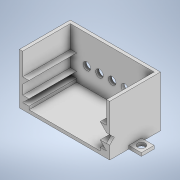
# Autodesk Inventor part: PCB_Case02
Saved by Autodesk Inventor 2021 (Build 250183000, 183)
## iProperties
Created: 2021-02-15
Part Number: PCB_Case02
Material: Generic
Document SubType Name: Modeling
Designer: Ryan
Density: 1 g/cm^3
Appearance: Default
Author: Ryan
Autodesk Inventor part; units mm, degrees
ref_plane "YZ Plane" through (0, 0, 0) normal (1, 0, 0) x (0, 1, 0)
ref_plane "XZ Plane" through (0, 0, 0) normal (0, 1, 0) x (-1, 0, 0)
ref_plane "XY Plane" through (0, 0, 0) normal (0, 0, 1) x (1, 0, 0)
sketch "Sketch1" plane through (0, 0, 0) normal (0, 1, 0) x (-1, 0, 0)
  line L0 (45.085, 25.4) -> (-45.085, 25.4)
  line L1 (-45.085, 25.4) -> (-45.085, -25.4)
  line L2 (-45.085, -25.4) -> (45.085, -25.4)
  line L3 (45.085, -25.4) -> (45.085, 25.4)
  point P0 (0, 0)
  dimension "d0" = 90.17
  dimension "d1" = 45.085
  dimension "d2" = 50.8
  dimension "d3" = 25.4
  constraints: 8 end point, 2 parallel, 1 horizontal, 1 perpendicular
  measures "d0" distance of L0.start L0.end
  measures "d1" distance from line of point (0, 0) L3
  measures "d2" distance of L0.end L1.end
  measures "d3" distance from line of point (0, 0) L2
extrude "Extrusion1" add sketch "Sketch1" along normal blind 50.8
sketch "Sketch2" plane through (0, 0, 0) normal (0, 1, 0) x (-1, 0, 0)
  line L0 (45.085, -25.4) -> (45.085, 25.4) projected
  line L1 (45.085, 6.35) -> (57.785, 6.35)
  line L2 (57.785, 6.35) -> (57.785, -6.35)
  line L3 (57.785, -6.35) -> (45.085, -6.35)
  line L4 (45.085, -6.35) -> (45.085, 6.35)
  line L5 (-45.085, 25.4) -> (-45.085, -25.4) projected
  line L6 (-45.085, -6.35) -> (-57.785, -6.35)
  line L7 (-57.785, -6.35) -> (-57.785, 6.35)
  line L8 (-57.785, 6.35) -> (-45.085, 6.35)
  line L9 (-45.085, 6.35) -> (-45.085, -6.35)
  circle A0 centre (51.435, 0) radius 3.81
  circle A1 centre (-51.435, 0) radius 3.81
  line L10 (51.435, 0) -> (51.435, -6.35) construction
  point P0 (0, 0)
  point P1 (-45.085, 6.35)
  point P2 (45.085, -6.35)
  dimension "d6" = 12.7
  dimension "d7" = 12.7
  dimension "d8" = 6.35
  dimension "d9" = 7.62
  dimension "d34" = 6.35
  dimension "d35" = 6.35
  dimension "d37" = 6.35
  constraints: 18 end point, 4 parallel, 2 centre point, 2 equal length, 2 horizontal, 2 perpendicular, 2 point on line, 1 collinear, 1 equal radius, 1 midpoint
  measures "d6" distance of L7.end L8.end
  measures "d7" distance of L6.end L7.end
  measures "d8" distance from line of point (0, 0) L6
  measures "d9" diameter of A0
  measures "d34" distance from line of L7 A1.centre
  measures "d35" distance from line of L6 A1.centre
  measures "d37" distance from line of L2 L10.start
extrude "Extrusion2" add sketch "Sketch2" along normal blind 3.175
sketch "Sketch4" plane through (-45.085, 0, 25.4) normal (0, 0, 1) x (1, 0, 0)
  line L0 (9.525, 3.175) -> (80.645, 3.175)
  line L1 (90.17, 0) -> (90.17, 50.8) projected
  line L2 (0, 50.8) -> (90.17, 50.8) projected
  line L3 (0, 0) -> (90.17, 0) projected
  line L4 (3.175, 40.8121) -> (3.175, 50.8)
  line L5 (90.17, 50.8) -> (0, 50.8) projected
  circle A0 centre (13.335, 40.8121) radius 2.5681 construction
  circle A1 centre (29.21, 40.8121) radius 2.5681 construction
  circle A2 centre (45.085, 40.8121) radius 2.6318 construction
  circle A3 centre (60.96, 40.8121) radius 2.9599 construction
  circle A4 centre (76.835, 40.8121) radius 2.9663 construction
  line L6 (3.175, 40.8121) -> (13.335, 40.8121) construction
  line L7 (13.335, 40.8121) -> (29.21, 40.8121) construction
  line L8 (29.21, 40.8121) -> (45.085, 40.8121) construction
  line L9 (45.085, 40.8121) -> (60.96, 40.8121) construction
  line L10 (60.96, 40.8121) -> (76.835, 40.8121) construction
  line L11 (76.835, 40.8121) -> (86.995, 40.8121) construction
  line L12 (3.175, 6.35) -> (9.525, 12.7)
  line L13 (9.525, 12.7) -> (3.175, 12.7)
  line L14 (3.175, 22.225) -> (9.525, 28.575)
  line L15 (9.525, 28.575) -> (3.175, 28.575)
  line L16 (45.085, 3.175) -> (45.085, 50.8) construction
  line L17 (3.175, 22.225) -> (3.175, 12.7)
  line L18 (0, 0) -> (0, 50.8) projected
  line L19 (90.17, 0) -> (0, 0) projected
  line L20 (3.175, 6.35) -> (9.525, 6.35)
  line L21 (9.525, 6.35) -> (9.525, 3.175)
  line L22 (86.995, 6.35) -> (80.645, 6.35)
  line L23 (80.645, 6.35) -> (80.645, 3.175)
  line L24 (3.175, 28.575) -> (3.175, 40.8121)
  line L25 (86.995, 12.7) -> (86.995, 6.35)
  line L26 (86.995, 6.35) -> (80.645, 12.7)
  line L27 (80.645, 12.7) -> (86.995, 12.7)
  line L28 (86.995, 22.225) -> (80.645, 28.575)
  line L29 (80.645, 28.575) -> (86.995, 28.575)
  line L30 (86.995, 22.225) -> (86.995, 12.7)
  line L31 (86.995, 28.575) -> (86.995, 40.8121)
  line L32 (86.995, 40.8121) -> (86.995, 50.8)
  line L33 (90.17, 0) -> (90.17, 50.8) projected
  point P0 (45.085, 0)
  point P1 (3.175, 6.35)
  dimension "d15" = 3.175
  dimension "d19" = 15.875
  dimension "d22" = 6.35
  dimension "d23" = 9.525
  dimension "d25" = 6.35
  dimension "d26" = 25.4
  dimension "d39" = 6.35
  dimension "d40" = 6.35
  dimension "d41" = 3.175
  dimension "d42" = 3.175
  constraints: 54 end point, 9 collinear, 6 perpendicular, 5 centre point, 5 symmetric about line, 3 horizontal, 3 point on line, 2 midpoint, 2 parallel
  measures "d15" distance between parallel lines of L3 L0
  measures "d19" distance of L6.end L7.end
  measures "d22" distance of L13.end L12.end
  measures "d23" distance between parallel lines of L0 L13
  measures "d25" distance of L14.end L15.end
  measures "d26" distance between parallel lines of L0 L15
  measures "d39" distance of L20.start L20.end
  measures "d40" distance of L22.start L22.end
  measures "d41" distance of L0.start L20.end
  measures "d42" distance of L0.end L22.end
extrude "Extrusion3" cut sketch "Sketch4" against normal blind 47.625 contours L21 L20 L12 L13 L17 L14 L15 L24 L4 L2 L32 L31 L29 L28 L30 L27 L26 L22 L23 L0
sketch "Sketch5" plane through (-45.085, 0, -22.225) normal (0, 0, 1) x (1, 0, 0)
  line L0 (3.175, 12.065) -> (3.175, 22.225) projected
  line L1 (19.7358, 22.225) -> (32.4104, 22.225) construction
  line L2 (32.4104, 22.225) -> (45.085, 22.225) construction
  line L3 (45.085, 22.225) -> (57.7596, 22.225) construction
  line L4 (57.7596, 22.225) -> (70.4342, 22.225) construction
  line L5 (86.995, 22.225) -> (86.995, 12.065) projected
  circle A0 centre (19.7358, 22.225) radius 3.81
  circle A1 centre (32.4104, 22.225) radius 3.81
  circle A2 centre (45.085, 22.225) radius 3.81
  circle A3 centre (57.7596, 22.225) radius 3.81
  circle A4 centre (70.4342, 22.225) radius 3.81
  line L6 (19.7358, 22.225) -> (3.175, 22.225) construction
  line L7 (70.4342, 22.225) -> (86.995, 22.225) construction
  line L8 (80.645, 3.175) -> (9.525, 3.175) projected
  line L9 (0, 0) -> (90.17, 0) projected
  point P0 (45.085, 0)
  point P1 (86.995, 3.175)
  point P2 (3.175, 3.175)
  dimension "d29" = 12.6746
  dimension "d30" = 7.62
  dimension "d38" = 22.225
  constraints: 12 end point, 6 collinear, 5 centre point, 5 coincident, 5 point on line, 4 equal radius
  measures "d29" distance of L1.start L1.end
  measures "d30" diameter of A0
  measures "d38" distance between parallel lines of L9 L2
extrude "Extrusion4" cut sketch "Sketch5" against normal blind 47.625
sketch "Sketch7" plane through (0, 0, 0) normal (1, 0, 0) x (0, 1, 0)
  line L0 (0, -25.4) -> (50.8, -25.4) projected
  line L1 (50.8, -25.4) -> (47.625, -25.4)
  line L2 (47.625, -25.4) -> (42.545, -24.13)
  line L3 (42.545, -24.13) -> (37.465, -25.4)
  line L4 (37.465, -25.4) -> (47.625, -25.4)
  line L5 (50.8, 25.4) -> (50.8, -25.4) projected
  point P0 (0, 0)
  point P1 (37.465, -25.4)
  dimension "d43" = 3.175
  dimension "d44" = 1.27
  dimension "d45" = 10.16
  constraints: 8 end point, 2 point on line, 1 collinear, 1 equal length
  measures "d43" distance from line of L5 L1.end
  measures "d44" distance from line of L2.end L4
  measures "d45" distance of L3.end L1.end
extrude "Extrusion5" cut sketch "Sketch7" against normal mid plane 12.7
sketch "Sketch8" plane through (45.085, 0, -25.4) normal (1, 0, 0) x (0, 0, -1)
  line L0 (-50.8, 12.7) -> (-50.8, 12.8905) construction
  line L1 (-50.8, 0) -> (-50.8, 50.8) construction
  line L2 (-50.8, 12.8905) -> (-46.228, 17.4625)
  line L3 (-46.228, 17.4625) -> (-50.8, 22.0345)
  line L4 (-50.8, 22.0345) -> (-50.8, 22.225) construction
  line L5 (-50.8, 22.225) -> (-3.175, 22.225) construction
  line L6 (-50.8, 22.225) -> (-46.228, 22.225) construction
  line L7 (-46.228, 22.225) -> (-46.228, 17.4625) construction
  line L8 (-46.228, 17.4625) -> (-46.228, 12.7) construction
  line L9 (-50.8, 12.7) -> (-3.175, 12.7) construction
  line L10 (-46.228, 12.7) -> (-50.8, 12.7) construction
  line L11 (-50.8, 22.0345) -> (-50.8, 12.8905)
  point P0 (-25.4, 0)
  dimension "d48" = 45
  dimension "d49" = 45
  dimension "d50" = 4.572
  constraints: 18 end point, 5 point on line, 3 collinear, 2 perpendicular
  measures "d48" angle of L0 L2
  measures "d49" angle of L1 L3
  measures "d50" distance from line of L1 L2.end
extrude "Extrusion6" cut sketch "Sketch8" against normal blind 25.4
equation "\"d1\" = 0.5 * d0"
equation "\"d3\" = 0.5 * d2"
equation "\"d8\" = 0.5 * d7"
equation "\"d34\" = 0.5 * d6"
equation "\"d35\" = d34"
equation "\"d37\" = d8"
equation "\"d15\" = d12"
equation "\"d42\" = d41"
equation "\"d12\" = 3.175"
body "Solid1"
